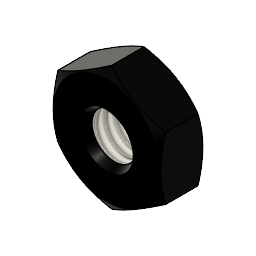
SBSPD (Autodesk Fusion 360 archive; units mm, degrees)
design "Hexagon Nut DIN 934 - M2.5 x 0.45 Stainless Steel A2-70 Black"
description: Hexagon Nut DIN 934 - M2.5 x 0.45
part number: DIN 934 - M2.5 x 0.45 Stainless Steel A2-70 Black
Autodesk Fusion 360 part; units mm, degrees
sketch "Sketch1" plane through (0, 0, 0) normal (0, 1, 0) x (1, 0, 0)
  line L0 (0, 0) -> (0, -2)
  line L1 (-1.25, 0) -> (-2.45, 0)
  line L2 (-2.45, 0) -> (-2.8875, -0.2526)
  line L3 (-2.8875, -0.2526) -> (-2.8875, -1.7474)
  line L4 (-2.8875, -1.7474) -> (-2.45, -2)
  line L5 (-2.45, -2) -> (-1.25, -2)
  line L6 (-1.25, -2) -> (-1.25, 0)
  dimension "d121" = 2.5
  dimension "d122" = 30
  dimension "d123" = 30
  dimension "d128" = 5.775
  dimension "d172" = 4.9
  dimension "d179" = 2
  constraint vertical L0
  constraint coincident L0 L0.end
  constraint coincident origin L0
  constraint horizontal L1
  constraint coincident L0.start L1
  constraint coincident L0.start origin
  constraint coincident L0.end L5
  constraint vertical L1.end L4.end
  measures "d122" angle of L1 L2
  measures "d123" angle of L4 L5
  measures "d179" distance of L1 L5
revolve "Revolve1" add sketch "Sketch1" angle 360 about axis through (0, 0, 0) along (0, 0, 1)
sketch "Sketch8" plane through (0, 0, 2) normal (0, 0, 1) x (1, 0, 0)
  line L0 (-2.5, -1.4449) -> (-2.5, 1.4449)
  circle A0 centre (0, 0) radius 1.25
  circle A1 centre (0, 0) radius 2.8875
  dimension "d114" = 2.5
  constraint coincident L0.end A1
  constraint coincident L0.start A1
  constraint vertical L0
  measures "d114" distance of A0.centre L0
extrude "Extrude5" cut sketch "Sketch8" against normal blind 2 contours L0 A1 picked at (-2.5625, 0.3519)
pattern_circular "C-Pattern2" count 6 over 360 about axis through (0, 0, 1.75) along (0, 0, 1) of "Extrude5"
thread "Thread3" "ISO Metric profile 2.5 M2.5x0.45 M2.5x0.45 6H" major diameter 2.58 minor diameter 2.0755 pitch 0.45 angle 60 resizes the face on face at (-1.2438, 0.1245, 1.3333)
sketch "Sketch12" plane through (0, 0, 0) normal (0, 1, 0) x (1, 0, 0)
  line L0 (-1.25, 0) -> (0, 0)
  line L1 (-0.6726, -1) -> (-1.25, 0)
  line L2 (-1.25, -2) -> (0, -2)
  line L3 (-0.6726, -1) -> (-1.25, -2)
  line L4 (0, 0) -> (0, -2)
  dimension "d169" = 60
  dimension "d177" = 1.25
  dimension "d178" = 60
  constraint horizontal L0
  constraint coincident L1.start L3.start
  constraint vertical L0.start L2.start
  constraint coincident L2.end L4.end
  constraint coincident L0.end L4.start
  constraint perpendicular L2 L4
  measures "d169" angle of L2 L3
  measures "d177" distance of L0.start L4
  measures "d178" angle of L0 L1
revolve "Revolve3" cut sketch "Sketch12" angle 360 about axis through (0, 0, 1.75) along (0, 0, 1)
equation "adsk_nheig = 2.00 mm"
equation "adsk_maxdia = 5.775 mm"
equation "adsk_nomdia = 2.50 mm"
equation "d89 = -adsk_nheig"
equation "adsk_waflat = 5.00 mm"
equation "d114 = adsk_waflat / 2"
equation "adsk_chamang1 = 30.00 deg"
equation "adsk_chamang2 = 30.00 deg"
equation "d121 = adsk_nomdia"
equation "d122 = adsk_chamang1"
equation "d123 = adsk_chamang2"
equation "d128 = adsk_maxdia"
equation "d163 = adsk_nheig"
equation "adsk_beardia = adsk_waflat * 0.98"
equation "d172 = adsk_beardia"
equation "d177 = adsk_nomdia * 0.5"
equation "d179 = adsk_nheig"

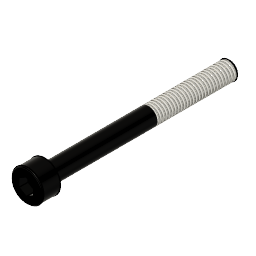
design "Hexagon Socket Head Cap Screw DIN EN ISO 4762 - M5 x 50 Steel 12.9 Black"
description: Hexagon Socket Head Cap Screw DIN EN ISO 4762 - M5 x 50
part number: DIN EN ISO 4762 - M5 x 50 Steel 12.9 Black
Autodesk Fusion 360 part; units mm, degrees
sketch "Sketch1" plane through (0, 0, 0) normal (0, 1, 0) x (1, 0, 0)
  line L0 (-2.5, 0) -> (-2.5, 50)
  line L1 (-2.5, 50) -> (0, 50)
  line L2 (0, 50) -> (0, -5)
  line L3 (-2.5, 0) -> (-4.25, 0)
  line L4 (-4.25, 0) -> (-4.25, -5)
  line L5 (-4.25, -5) -> (0, -5)
  dimension "d9" = 5
  dimension "d106" = 5
  dimension "d107" = 50
  dimension "d116" = 8.5
  constraint perpendicular L0 L1
  constraint collinear origin L1.end L2.end
  constraint perpendicular L0 L3
  constraint coincident origin L3
  constraint vertical L2
  constraint coincident L2 L5.end
  constraint perpendicular L2 L5
  measures "d106" distance of L3 L5
  measures "d107" distance of origin L1
revolve "Revolve1" add sketch "Sketch1" angle 360 about axis through (0, 0, -50) along (0, 0, 1)
ref_plane "WorkPlane1" through (0, 0, 5) normal (0, 0, 1) x (1, 0, 0)
sketch "Sketch6" plane through (0, 0, 5) normal (0, 0, 1) x (1, 0, 0)
  line L0 (-2, 1.1547) -> (-2, -1.1547)
  line L1 (-2, -1.1547) -> (0, -2.3094)
  line L2 (0, -2.3094) -> (2, -1.1547)
  line L3 (2, -1.1547) -> (2, 1.1547)
  line L4 (2, 1.1547) -> (0, 2.3094)
  line L5 (0, 2.3094) -> (-2, 1.1547)
  dimension "d117" = 4
  constraint vertical L0
  measures "d117" distance of L0 L3
extrude "Extrude1" cut sketch "Sketch6" against normal blind 2.5
extrude "Extrude2" cut 1 faces at (0.6667, -0.3849, 2.5) along direction (0, 0, -1) blind 2.5 draft -85
fillet "Fillet4" radius 0.5 1 edges at (-3.9624, 1.5369, 5)
thread "Thread3" "ISO Metric profile 5.0 M5x0.8 M5x0.8 6g" major diameter 4.901 minor diameter 3.9895 pitch 0.8 angle 60 resizes the face on face at (-2.4876, 0.2489, -33.3333) from (0, 0, -28) to (0, 0, -50)
sketch "Sketch7" plane through (0, 0, 0) normal (0, 1, 0) x (1, 0, 0)
  line L0 (-2.55, 50) -> (-2.55, 49.5)
  line L1 (-2.55, 49.5) -> (-2.05, 50)
  line L2 (0, 50) -> (0, -5)
  line L3 (-2.55, 50) -> (0, 50)
  dimension "d101" = 45
  dimension "d112" = 0.5
  dimension "d113" = 2.55
  constraint coincident L2.start L3.end
  constraint perpendicular L2 L3
  constraint coincident L1.end L3
  constraint perpendicular L0 L3
  measures "d101" angle of L0 L1
  measures "d112" distance of L0.end L3
  measures "d113" distance of L0 L2.start
revolve "Revolve3" cut sketch "Sketch7" angle 360 about axis through (0, 0, 1.75) along (0, 0, 1)
equation "d9 = adsk_nomdia"
equation "adsk_nomlen = 50.00 mm"
equation "adsk_headh = 5.00 mm"
equation "adsk_headdia = 8.50 mm"
equation "adsk_nomdia = 5.00 mm"
equation "adsk_philwidth = 4.00 mm"
equation "d31 = -adsk_phildepth"
equation "adsk_phildepth = 2.50 mm"
equation "d71 = adsk_headh"
equation "d76 = -adsk_phildepth"
equation "adsk_thrlen = 22.00 mm"
equation "d86 = adsk_nomdia * 0.1"
equation "adsk_startang = 45.00 deg"
equation "d101 = adsk_startang"
equation "adsk_pitch1 = 0.80 mm"
equation "adsk_startlen = 0.50 mm"
equation "d106 = adsk_headh"
equation "d107 = adsk_nomlen"
equation "d112 = adsk_startlen"
equation "d113 = adsk_nomdia * 0.51"
equation "d115 = min(adsk_thrlen; adsk_nomlen - 0.001 mm)"
equation "d116 = adsk_headdia"
equation "d117 = adsk_philwidth"

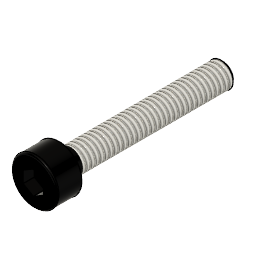
design "Hexagon Socket Head Cap Screw DIN EN ISO 4762 - M2.5 x 16 Steel 12.9 Black"
description: Hexagon Socket Head Cap Screw DIN EN ISO 4762 - M2.5 x 16
part number: DIN EN ISO 4762 - M2.5 x 16 Steel 12.9 Black
Autodesk Fusion 360 part; units mm, degrees
sketch "Sketch1" plane through (0, 0, 0) normal (0, 1, 0) x (1, 0, 0)
  line L0 (-1.25, 0) -> (-1.25, 16)
  line L1 (-1.25, 16) -> (0, 16)
  line L2 (0, 16) -> (0, -2.5)
  line L3 (-1.25, 0) -> (-2.25, 0)
  line L4 (-2.25, 0) -> (-2.25, -2.5)
  line L5 (-2.25, -2.5) -> (0, -2.5)
  dimension "d9" = 2.5
  dimension "d106" = 2.5
  dimension "d107" = 16
  dimension "d116" = 4.5
  constraint perpendicular L0 L1
  constraint collinear origin L1.end L2.end
  constraint perpendicular L0 L3
  constraint coincident origin L3
  constraint vertical L2
  constraint coincident L2 L5.end
  constraint perpendicular L2 L5
  measures "d106" distance of L3 L5
  measures "d107" distance of origin L1
revolve "Revolve1" add sketch "Sketch1" angle 360 about axis through (0, 0, -16) along (0, 0, 1)
ref_plane "WorkPlane1" through (0, 0, 2.5) normal (0, 0, 1) x (1, 0, 0)
sketch "Sketch6" plane through (0, 0, 2.5) normal (0, 0, 1) x (1, 0, 0)
  line L0 (-1, 0.5774) -> (-1, -0.5774)
  line L1 (-1, -0.5774) -> (0, -1.1547)
  line L2 (0, -1.1547) -> (1, -0.5774)
  line L3 (1, -0.5774) -> (1, 0.5774)
  line L4 (1, 0.5774) -> (0, 1.1547)
  line L5 (0, 1.1547) -> (-1, 0.5774)
  dimension "d117" = 2
  constraint vertical L0
  measures "d117" distance of L0 L3
extrude "Extrude1" cut sketch "Sketch6" against normal blind 1.1
extrude "Extrude2" cut 1 faces at (-0.3333, 0.1925, 1.4) along direction (0, 0, -1) blind 1.1 draft -85
fillet "Fillet4" radius 0.25 1 edges at (-2.0977, 0.8136, 2.5)
thread "Thread3" "ISO Metric profile 2.5 M2.5x0.45 M2.5x0.45 6g" major diameter 2.43 minor diameter 1.9165 pitch 0.45 angle 60 resizes the face on face at (-1.2438, 0.1245, -10.6667) from (0, 0, -1.125) to (0, 0, -16)
sketch "Sketch7" plane through (0, 0, 0) normal (0, 1, 0) x (1, 0, 0)
  line L0 (-1.275, 16) -> (-1.275, 15.75)
  line L1 (-1.275, 15.75) -> (-1.025, 16)
  line L2 (0, 16) -> (0, -2.5)
  line L3 (-1.275, 16) -> (0, 16)
  dimension "d101" = 45
  dimension "d112" = 0.25
  dimension "d113" = 1.275
  constraint coincident L2.start L3.end
  constraint perpendicular L2 L3
  constraint coincident L1.end L3
  constraint perpendicular L0 L3
  measures "d101" angle of L0 L1
  measures "d112" distance of L0.end L3
  measures "d113" distance of L0 L2.start
revolve "Revolve3" cut sketch "Sketch7" angle 360 about axis through (0, 0, 1.75) along (0, 0, 1)
equation "d9 = adsk_nomdia"
equation "adsk_nomlen = 16.00 mm"
equation "adsk_headh = 2.50 mm"
equation "adsk_headdia = 4.50 mm"
equation "adsk_nomdia = 2.50 mm"
equation "adsk_philwidth = 2.00 mm"
equation "d31 = -adsk_phildepth"
equation "adsk_phildepth = 1.10 mm"
equation "d71 = adsk_headh"
equation "d76 = -adsk_phildepth"
equation "adsk_thrlen = 14.875 mm"
equation "d86 = adsk_nomdia * 0.1"
equation "adsk_startang = 45.00 deg"
equation "d101 = adsk_startang"
equation "adsk_pitch1 = 0.45 mm"
equation "adsk_startlen = 0.25 mm"
equation "d106 = adsk_headh"
equation "d107 = adsk_nomlen"
equation "d112 = adsk_startlen"
equation "d113 = adsk_nomdia * 0.51"
equation "d115 = min(adsk_thrlen; adsk_nomlen - 0.001 mm)"
equation "d116 = adsk_headdia"
equation "d117 = adsk_philwidth"

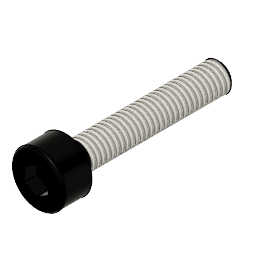
design "Hexagon Socket Head Cap Screw DIN EN ISO 4762 - M3 x 16 Steel 12.9 Black"
description: Hexagon Socket Head Cap Screw DIN EN ISO 4762 - M3 x 16
part number: DIN EN ISO 4762 - M3 x 16 Steel 12.9 Black
Autodesk Fusion 360 part; units mm, degrees
sketch "Sketch1" plane through (0, 0, 0) normal (0, 1, 0) x (1, 0, 0)
  line L0 (-1.5, 0) -> (-1.5, 16)
  line L1 (-1.5, 16) -> (0, 16)
  line L2 (0, 16) -> (0, -3)
  line L3 (-1.5, 0) -> (-2.75, 0)
  line L4 (-2.75, 0) -> (-2.75, -3)
  line L5 (-2.75, -3) -> (0, -3)
  dimension "d9" = 3
  dimension "d106" = 3
  dimension "d107" = 16
  dimension "d116" = 5.5
  constraint perpendicular L0 L1
  constraint collinear origin L1.end L2.end
  constraint perpendicular L0 L3
  constraint coincident origin L3
  constraint vertical L2
  constraint coincident L2 L5.end
  constraint perpendicular L2 L5
  measures "d106" distance of L3 L5
  measures "d107" distance of origin L1
revolve "Revolve1" add sketch "Sketch1" angle 360 about axis through (0, 0, -16) along (0, 0, 1)
ref_plane "WorkPlane1" through (0, 0, 3) normal (0, 0, 1) x (1, 0, 0)
sketch "Sketch6" plane through (0, 0, 3) normal (0, 0, 1) x (1, 0, 0)
  line L0 (-1.25, 0.7217) -> (-1.25, -0.7217)
  line L1 (-1.25, -0.7217) -> (0, -1.4434)
  line L2 (0, -1.4434) -> (1.25, -0.7217)
  line L3 (1.25, -0.7217) -> (1.25, 0.7217)
  line L4 (1.25, 0.7217) -> (0, 1.4434)
  line L5 (0, 1.4434) -> (-1.25, 0.7217)
  dimension "d117" = 2.5
  constraint vertical L0
  measures "d117" distance of L0 L3
extrude "Extrude1" cut sketch "Sketch6" against normal blind 1.3
extrude "Extrude2" cut 1 faces at (0.4167, 0.2406, 1.7) along direction (0, 0, -1) blind 1.3 draft -85
fillet "Fillet4" radius 0.3 1 edges at (-2.5639, 0.9944, 3)
thread "Thread3" "ISO Metric profile 3.0 M3x0.5 M3x0.5 6g" major diameter 2.927 minor diameter 2.3555 pitch 0.5 angle 60 resizes the face on face at (-1.4925, 0.1494, -10.6667) from (0, 0, -1.25) to (0, 0, -16)
sketch "Sketch7" plane through (0, 0, 0) normal (0, 1, 0) x (1, 0, 0)
  line L0 (-1.53, 16) -> (-1.53, 15.7)
  line L1 (-1.53, 15.7) -> (-1.23, 16)
  line L2 (0, 16) -> (0, -3)
  line L3 (-1.53, 16) -> (0, 16)
  dimension "d101" = 45
  dimension "d112" = 0.3
  dimension "d113" = 1.53
  constraint coincident L2.start L3.end
  constraint perpendicular L2 L3
  constraint coincident L1.end L3
  constraint perpendicular L0 L3
  measures "d101" angle of L0 L1
  measures "d112" distance of L0.end L3
  measures "d113" distance of L0 L2.start
revolve "Revolve3" cut sketch "Sketch7" angle 360 about axis through (0, 0, 1.75) along (0, 0, 1)
equation "d9 = adsk_nomdia"
equation "adsk_nomlen = 16.00 mm"
equation "adsk_headh = 3.00 mm"
equation "adsk_headdia = 5.50 mm"
equation "adsk_nomdia = 3.00 mm"
equation "adsk_philwidth = 2.50 mm"
equation "d31 = -adsk_phildepth"
equation "adsk_phildepth = 1.30 mm"
equation "d71 = adsk_headh"
equation "d76 = -adsk_phildepth"
equation "adsk_thrlen = 14.75 mm"
equation "d86 = adsk_nomdia * 0.1"
equation "adsk_startang = 45.00 deg"
equation "d101 = adsk_startang"
equation "adsk_pitch1 = 0.50 mm"
equation "adsk_startlen = 0.30 mm"
equation "d106 = adsk_headh"
equation "d107 = adsk_nomlen"
equation "d112 = adsk_startlen"
equation "d113 = adsk_nomdia * 0.51"
equation "d115 = min(adsk_thrlen; adsk_nomlen - 0.001 mm)"
equation "d116 = adsk_headdia"
equation "d117 = adsk_philwidth"

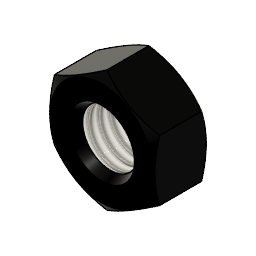
design "Hexagon Nut DIN 934 - M5 x 0.8 Stainless Steel A2-70 Black"
description: Hexagon Nut DIN 934 - M5 x 0.8
part number: DIN 934 - M5 x 0.8 Stainless Steel A2-70 Black
Autodesk Fusion 360 part; units mm, degrees
sketch "Sketch1" plane through (0, 0, 0) normal (0, 1, 0) x (1, 0, 0)
  line L0 (0, 0) -> (0, -4)
  line L1 (-2.5, 0) -> (-3.92, 0)
  line L2 (-3.92, 0) -> (-4.62, -0.4041)
  line L3 (-4.62, -0.4041) -> (-4.62, -3.5959)
  line L4 (-4.62, -3.5959) -> (-3.92, -4)
  line L5 (-3.92, -4) -> (-2.5, -4)
  line L6 (-2.5, -4) -> (-2.5, 0)
  dimension "d121" = 5
  dimension "d122" = 30
  dimension "d123" = 30
  dimension "d128" = 9.24
  dimension "d172" = 7.84
  dimension "d179" = 4
  constraint vertical L0
  constraint coincident L0 L0.end
  constraint coincident origin L0
  constraint horizontal L1
  constraint coincident L0.start L1
  constraint coincident L0.start origin
  constraint coincident L0.end L5
  constraint vertical L1.end L4.end
  measures "d122" angle of L1 L2
  measures "d123" angle of L4 L5
  measures "d179" distance of L1 L5
revolve "Revolve1" add sketch "Sketch1" angle 360 about axis through (0, 0, 0) along (0, 0, 1)
sketch "Sketch8" plane through (0, 0, 4) normal (0, 0, 1) x (1, 0, 0)
  line L0 (-4, -2.3118) -> (-4, 2.3118)
  circle A0 centre (0, 0) radius 2.5
  circle A1 centre (0, 0) radius 4.62
  dimension "d114" = 4
  constraint coincident L0.end A1
  constraint coincident L0.start A1
  constraint vertical L0
  measures "d114" distance of A0.centre L0
extrude "Extrude5" cut sketch "Sketch8" against normal blind 4 contours L0 A1 picked at (-4.1, -0.5631)
pattern_circular "C-Pattern2" count 6 over 360 about axis through (0, 0, 1.75) along (0, 0, 1) of "Extrude5"
thread "Thread3" "ISO Metric profile 5.0 M5x0.8 M5x0.8 6H" major diameter 5.12 minor diameter 4.234 pitch 0.8 angle 60 resizes the face on face at (-2.4876, 0.2489, 2.6667)
sketch "Sketch12" plane through (0, 0, 0) normal (0, 1, 0) x (1, 0, 0)
  line L0 (-2.5, 0) -> (0, 0)
  line L1 (-1.3453, -2) -> (-2.5, 0)
  line L2 (-2.5, -4) -> (0, -4)
  line L3 (-1.3453, -2) -> (-2.5, -4)
  line L4 (0, 0) -> (0, -4)
  dimension "d169" = 60
  dimension "d177" = 2.5
  dimension "d178" = 60
  constraint horizontal L0
  constraint coincident L1.start L3.start
  constraint vertical L0.start L2.start
  constraint coincident L2.end L4.end
  constraint coincident L0.end L4.start
  constraint perpendicular L2 L4
  measures "d169" angle of L2 L3
  measures "d177" distance of L0.start L4
  measures "d178" angle of L0 L1
revolve "Revolve3" cut sketch "Sketch12" angle 360 about axis through (0, 0, 1.75) along (0, 0, 1)
equation "adsk_nheig = 4.00 mm"
equation "adsk_maxdia = 9.24 mm"
equation "adsk_nomdia = 5.00 mm"
equation "d89 = -adsk_nheig"
equation "adsk_waflat = 8.00 mm"
equation "d114 = adsk_waflat / 2"
equation "adsk_chamang1 = 30.00 deg"
equation "adsk_chamang2 = 30.00 deg"
equation "d121 = adsk_nomdia"
equation "d122 = adsk_chamang1"
equation "d123 = adsk_chamang2"
equation "d128 = adsk_maxdia"
equation "d163 = adsk_nheig"
equation "adsk_beardia = adsk_waflat * 0.98"
equation "d172 = adsk_beardia"
equation "d177 = adsk_nomdia * 0.5"
equation "d179 = adsk_nheig"
